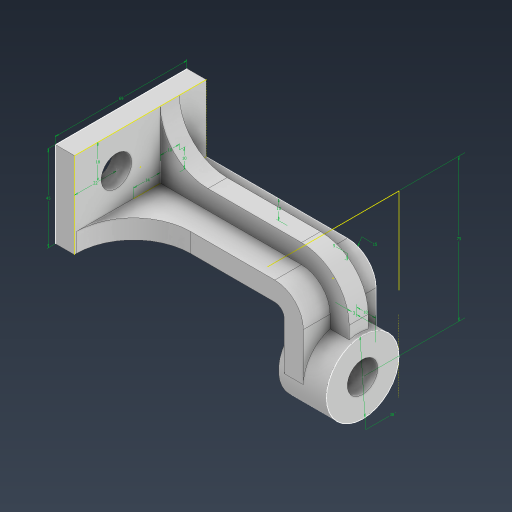
# Autodesk Inventor part: Peça teste 6
Saved by Autodesk Inventor 2024 (Build 280153000, 153)
## iProperties
Created: 2024-02-13
Part Number: Peça teste 6
Material: Genérico
Document SubType Name: Modeling
Designer: Administrator
Density: 1 g/cm^3
Appearance: Padrão
Author: Administrator
Autodesk Inventor part; units mm, degrees
ref_plane "YZ Plane" through (0, 0, 0) normal (1, 0, 0) x (0, 1, 0)
ref_plane "XZ Plane" through (0, 0, 0) normal (0, 1, 0) x (-1, 0, 0)
sketch "Esboço1" plane through (0, 0, 0) normal (1, 0, 0) x (0, 1, 0)
  line L0 (-22.5, -34.5) -> (22.5, -34.5)
  line L1 (22.5, -34.5) -> (22.5, 34.5)
  line L2 (22.5, 34.5) -> (-22.5, 34.5)
  line L3 (-22.5, 34.5) -> (-22.5, -34.5)
  line L4 (-22.5, -34.5) -> (22.5, 34.5) construction
  line L5 (22.5, -34.5) -> (-22.5, 34.5) construction
  point P0 (0, 0)
  dimension "d0" = 45
  dimension "d1" = 69
  constraints: 12 end point, 2 midpoint, 2 parallel, 1 horizontal, 1 perpendicular
  measures "d0" distance of L2.end L1.end
  measures "d1" distance of L1.end L0.end
extrude "Extrusão1" add sketch "Esboço1" along normal blind 10
sketch "Esboço2" plane through (10, 0, 0) normal (1, 0, 0) x (0, 0, -1)
  line L0 (34.5, 22.5) -> (-34.5, 22.5) projected
  line L1 (-34.5, 22.5) -> (-34.5, -22.5) projected
  point P0 (0, 0)
  point P1 (-12.5, 4.5)
  dimension "d4" = 18
  dimension "d5" = 22
  measures "d4" distance from line of L0 point (-12.5, 4.5)
  measures "d5" distance from line of L1 point (-12.5, 4.5)
hole "Furo1" at (10, 4.5, 12.5) direction (-1, 0, 0) diameter 16 end through all
ref_plane "Plano de trabalho1" through (111, 0, 0) normal (1, 0, 0) x (0, 0, -1)
sketch "Esboço3" plane through (111, 0, 0) normal (1, 0, 0) x (0, 0, -1)
  circle A0 centre (15.5, -52.5) radius 19
  line L0 (34.5, -22.5) -> (34.5, 22.5) projected
  line L1 (34.5, 22.5) -> (-34.5, 22.5) projected
  point P0 (0, 0)
  dimension "d14" = 38
  dimension "d15" = 75
  constraints: 1 centre point, 1 tangent
  measures "d14" diameter of A0
  measures "d15" distance from line of A0.centre L1
extrude "Extrusão2" add sketch "Esboço3" against normal blind 25
sketch "Esboço5" plane through (0, -22.5, -34.5) normal (0, 0, -1) x (-1, 0, 0)
  line L0 (-10, 45) -> (-10, 0) construction
  line L1 (-10, 0) -> (-84, 0)
  line L2 (-89, -5) -> (-89, -30)
  line L3 (-89, -30) -> (-99, -30)
  line L4 (-99, -30) -> (-99, -5)
  line L5 (-84, 10) -> (-10, 10)
  line L6 (-111, -11) -> (-111, -49) construction
  line L7 (-111, -30) -> (-86, -30) construction
  line L8 (-86, -49) -> (-86, -11) construction
  arc A0 (-84, 0) -> (-89, -5) centre (-84, -5) ccw
  arc A1 (-84, 10) -> (-99, -5) centre (-84, -5) ccw
  point P0 (0, 22.5)
  dimension "d18" = 3
  dimension "d19" = 10
  dimension "d20" = 10
  dimension "d21" = 5
  dimension "d22" = 15
  constraints: 12 end point, 4 perpendicular, 4 point on circle, 4 tangent, 2 centre point, 2 midpoint, 2 point on line, 1 horizontal
  measures "d18" distance between parallel lines of L8 L2
  measures "d19" distance between parallel lines of L2 L4
  measures "d20" distance between parallel lines of L5 L1
  measures "d21" radius of A0
  measures "d22" radius of A1
extrude "Extrusão3" add sketch "Esboço5" against normal blind 38 fills toward (-47, 0.05) open curves L1 A0 L2 L3 L4 A1 L5
sketch "Esboço6" plane through (10, 0, 0) normal (1, 0, 0) x (0, 0, -1)
  line L0 (34.5, -12.5) -> (-3.5, -12.5) projected
  line L1 (10.5, -12.5) -> (20.5, -12.5)
  line L2 (20.5, -12.5) -> (20.5, -2.5)
  line L3 (20.5, -2.5) -> (10.5, -2.5)
  line L4 (10.5, -2.5) -> (10.5, -12.5)
  line L5 (-3.5, -12.5) -> (-3.5, -27.5) projected
  point P0 (0, 0)
  dimension "d26" = 10
  dimension "d27" = 10
  dimension "d28" = 14
  constraints: 8 end point, 2 parallel, 1 horizontal, 1 perpendicular, 1 point on line
  measures "d26" distance of L3.end L2.end
  measures "d27" distance of L2.end L1.end
  measures "d28" distance between parallel lines of L4 L5
sketch3d "Esboço 3D1"
  line L0 (10, -12.5, -34.5) -> (84, -12.5, -34.5)
  arc A0 (84, -12.5, -34.5) -> (99, -27.5, -34.5) centre (84, -27.5, -34.5) ccw
  line L1 (99, -27.5, -34.5) -> (99, -52.5, -34.5)
sweep "Varredura1" add profiles "Esboço6" path "Esboço 3D1"
sketch "Esboço7" plane through (111, -52.5, -15.5) normal (1, 0, 0) x (0, 0, -1)
  circle A0 centre (0, 0) radius 19 projected
  point P0 (-15.5, 52.5)
  constraints: 1 coincident
hole "Furo2" at (111, -52.5, -15.5) direction (-1, 0, 0) diameter 16 end through all
fillet "Arredondamento1" radius 25 1 edges at (10, -2.5, -15.5)
fillet "Arredondamento2" radius 30 1 edges at (10, -17.5, 3.5)
